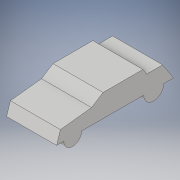
# Autodesk Inventor part: car110th
Saved by Autodesk Inventor 2019 (Build 230136000, 136)
## iProperties
Created: 2020-04-29
Part Number: car110th
Material: Generic
Document SubType Name: Modeling
Designer: infinity
Density: 1 g/cm^3
Appearance: Default
Author: infinity
Autodesk Inventor part; units mm, degrees
ref_plane "YZ Plane" through (0, 0, 0) normal (1, 0, 0) x (0, 1, 0)
ref_plane "XZ Plane" through (0, 0, 0) normal (0, 1, 0) x (-1, 0, 0)
ref_plane "XY Plane" through (0, 0, 0) normal (0, 0, 1) x (1, 0, 0)
sketch "Sketch1" plane through (0, 0, 0) normal (1, 0, 0) x (0, 1, 0)
  line L0 (0, 0) -> (0, -280)
  line L1 (0, 0) -> (28.1328, -9.1597)
  line L2 (28.1328, -9.1597) -> (36.7239, -83.6155)
  line L3 (36.7239, -83.6155) -> (54.1655, -111.3657)
  line L4 (54.1655, -111.3657) -> (54.1655, -206.8716)
  line L5 (54.1655, -206.8716) -> (40.2194, -215.637)
  line L6 (40.2194, -215.637) -> (40.2194, -254.0323)
  line L7 (40.2194, -254.0323) -> (0, -280)
  dimension "d0" = 280
  dimension "d2" = 0
  constraints: 16 end point, 1 coincident, 1 parallel, 1 perpendicular, 1 vertical
  measures "d0" distance of L0.start L0.end
  measures "d2" horizontal distance of L0.start L0.end
extrude "Extrusion1" add sketch "Sketch1" along normal blind 120
sketch "Sketch2" plane through (120, 0, 0) normal (1, 0, 0) x (0, 0, -1)
  line L0 (0, 0) -> (280, 0) projected
  circle A0 centre (38.4586, 0) radius 21.4935
  circle A1 centre (232.7073, 0) radius 24.1819
  constraints: 2 centre point, 2 point on line
extrude "Extrusion2" add sketch "Sketch2" against normal blind 120
body "Solid1"
